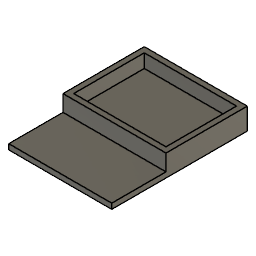
MOSFET_Halterung (Autodesk Fusion 360 design; units mm, degrees)
Autodesk Fusion 360 part; units mm, degrees
box "Grundkörper Quader1" add length 30 width 38 height 2 placed x (0, -1, 0) y (1, 0, 0) z (0, 0, 1) at (0, 0, 0) makes body 1
box "Grundkörper Quader2" add length 30 width 38 height 5 placed x (0, -1, 0) y (1, 0, 0) z (0, 0, 1) at (0, 0, 2) separate body makes body 2
shell "Schale1" thickness 2 removed faces 2 at (25.3333, -10, 7) at (25.3333, -10, 2) on bodies 2
extrude "Extrusion1" add 1 faces at (12.6667, -30, 0.6667) along direction (0, -1, 0) blind 20 on bodies 1 bodies 1 2
extrude "Extrusion2" add 1 faces at (24.6667, -10.6667, 2) along direction (0, 0, 1) blind 1 on bodies 1 bodies 1
extrude "Extrusion3" add 1 faces at (13.3333, -0.6667, 7) along direction (0, 0, 1) blind 1 on bodies 1 bodies 1
